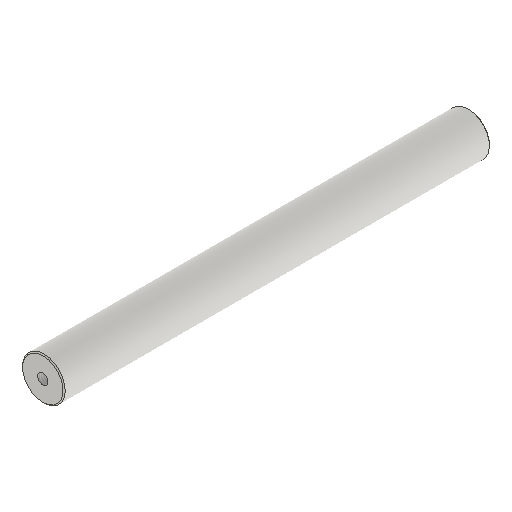
# Autodesk Inventor part: DLT-01-236B
Saved by Autodesk Inventor 2025.2 (Build 292293000, 293)
## iProperties
Company: Delta
Created: 2024-10-21
Part Number: DLT-01-236B
Material: Aço SAE 1045
Document SubType Name: Modeling
Designer: Willian Pinheiro
Density: 7.85 g/cm^3
Appearance: Steel
Description: Eixo Guia Pressor B
Mass: 490.054 g
Surface Area: 134.693 cm^2
Volume: 62.4273 cm^3
Project: DLT
Dimensões: Ø20 x 200 mm
Total: 2
Author: Willian Pinheiro
Revision Number: 00
Autodesk Inventor part; units mm, degrees
ref_plane "YZ Plane" through (0, 0, 0) normal (1, 0, 0) x (0, 1, 0)
ref_plane "XZ Plane" through (0, 0, 0) normal (0, 1, 0) x (-1, 0, 0)
ref_plane "XY Plane" through (0, 0, 0) normal (0, 0, 1) x (1, 0, 0)
sketch "Sketch1" plane through (0, 0, 0) normal (1, 0, 0) x (0, 1, 0)
  line L0 (-140, 0) -> (140, 0) construction
  line L1 (0, -2) -> (0, 12) construction
  line L2 (-100, 10) -> (100, 10)
  line L3 (100, 10) -> (100, 0)
  line L4 (100, 0) -> (-100, 0)
  line L5 (-100, 0) -> (-100, 10)
  point P0 (0, 0)
  dimension "d0" = 20
  dimension "d1" = 200
  constraints: 8 end point, 2 parallel, 1 horizontal, 1 perpendicular, 1 point on line, 1 other
  measures "d0" diameter of L2 L0
  measures "d1" distance of L2.start L2.end
revolve "Revolution1" add sketch "Sketch1" angle 360 about axis through (0, -10, 0) along (0, 1, 0)
sketch "Sketch2" plane through (0, -100, 0) normal (0, -1, 0) x (1, 0, 0)
  circle A0 centre (0, 0) radius 10 projected
  constraints: 1 coincident
hole "Hole1" at (0, -100, 0) direction (0, 1, 0) diameter 4.917 depth 20 tip angle 118 thread size "M6x1" class "6H" standard "ISO Metric profile"
chamfer "Chamfer1" distance 0.5 angle 45 2 edges at (0, -100, -10) (0, 100, -10)
body "Solid1"
